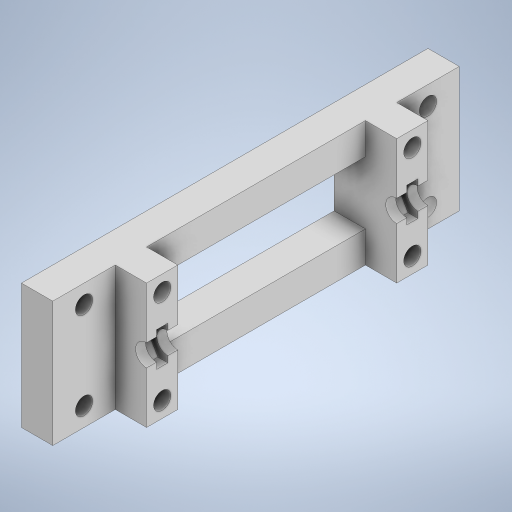
# Autodesk Inventor part: MotorDifferentialMountingBracket
Saved by Autodesk Inventor 2023 (Build 270158000, 158)
## iProperties
Created: 2023-03-28
Part Number: MotorDifferentialMountingBracket
Material: Generic
Document SubType Name: Modeling
Designer: Nathann
Density: 1 g/cm^3
Appearance: Default
Author: Nathann
Autodesk Inventor part; units mm, degrees
ref_plane "YZ Plane" through (0, 0, 0) normal (1, 0, 0) x (0, 1, 0)
ref_plane "XZ Plane" through (0, 0, 0) normal (0, 1, 0) x (-1, 0, 0)
ref_plane "XY Plane" through (0, 0, 0) normal (0, 0, 1) x (1, 0, 0)
sketch "Sketch1" plane through (0, 0, 0) normal (0, 1, 0) x (-1, 0, 0)
  line L0 (0, 0) -> (-5, 0)
  line L1 (-5, 0) -> (-5, 45)
  line L2 (-5, 45) -> (0, 45)
  line L3 (0, 45) -> (0, 0)
  line L4 (-5, 45) -> (-20, 45)
  line L5 (-20, 45) -> (-20, 40)
  line L6 (-20, 40) -> (-5, 40)
  line L7 (-5, 40) -> (-5, 45)
  line L8 (-5, 0) -> (-20, 0)
  line L9 (-20, 0) -> (-20, 5)
  line L10 (-20, 5) -> (-5, 5)
  line L11 (-5, 5) -> (-5, 0)
  point P0 (-5, 40)
  point P1 (-5, 5)
  dimension "d0" = 5
  dimension "d1" = 5
  dimension "d2" = 5
  dimension "d3" = 15
  dimension "d4" = 15
  dimension "d5" = 35
  constraints: 24 end point, 6 parallel, 3 horizontal, 3 perpendicular, 1 point on line
  measures "d0" distance between parallel lines of L3 L1
  measures "d1" distance between parallel lines of L6 L4
  measures "d2" distance between parallel lines of L8 L10
  measures "d3" distance between parallel lines of L5 L1
  measures "d4" distance between parallel lines of L1 L9
  measures "d5" distance between parallel lines of L10 L6
extrude "Extrusion1" add sketch "Sketch1" along normal blind 20
sketch "Sketch2" plane through (0, 0, 45) normal (0, 0, 1) x (1, 0, 0)
  circle A0 centre (10, 10) radius 1.75
  line L0 (20, 0) -> (20, 20) projected
  line L1 (20, 0) -> (10, 0)
  line L2 (10, 0) -> (10, 20)
  line L3 (10, 20) -> (20, 20)
  line L4 (20, 20) -> (20, 0)
  line L5 (0, 0) -> (20, 0) projected
  dimension "d8" = 10
  dimension "d9" = 10
  dimension "d10" = 10
  dimension "d11" = 3.5
  constraints: 8 end point, 2 parallel, 1 centre point, 1 horizontal, 1 perpendicular
  measures "d8" distance between parallel lines of L0 L2
  measures "d9" distance from line of L0 A0.centre
  measures "d10" distance from line of L5 A0.centre
  measures "d11" diameter of A0
extrude "Extrusion2" cut sketch "Sketch2" against normal blind 200
sketch "Sketch3" plane through (0, 0, 0) normal (-1, 0, 0) x (0, 0, 1)
  line L0 (5, 0) -> (5, 20) projected
  line L1 (40, 0) -> (40, 20) projected
  line L2 (5, 15) -> (40, 15)
  line L3 (40, 15) -> (40, 5)
  line L4 (40, 5) -> (5, 5)
  line L5 (5, 5) -> (5, 15)
  line L6 (0, 20) -> (45, 20) projected
  line L7 (0, 0) -> (45, 0) projected
  point P0 (5, 5)
  dimension "d14" = 5
  dimension "d15" = 5
  constraints: 8 end point, 2 parallel, 2 point on line, 1 horizontal, 1 perpendicular
  measures "d14" distance between parallel lines of L6 L2
  measures "d15" distance between parallel lines of L7 L4
extrude "Extrusion3" cut sketch "Sketch3" against normal blind 20 contours L0 L2 L1 L4
sketch "Sketch4" plane through (0, 0, 0) normal (-1, 0, 0) x (0, 0, 1)
  line L0 (45, 0) -> (45, 20) projected
  line L1 (45, 20) -> (55, 20)
  line L2 (55, 20) -> (55, 0)
  line L3 (55, 0) -> (45, 0)
  line L4 (45, 0) -> (45, 20)
  line L5 (0, 20) -> (0, 11.75) projected
  line L6 (0, 20) -> (-10, 20)
  line L7 (-10, 20) -> (-10, 0)
  line L8 (-10, 0) -> (0, 0)
  line L9 (0, 0) -> (0, 20)
  circle A0 centre (50, 3) radius 1.375
  circle A1 centre (50, 17) radius 1.375
  circle A2 centre (-5, 17) radius 1.375
  circle A3 centre (-5, 3) radius 1.375
  point P0 (0, 0)
  point P1 (50, 20)
  dimension "d18" = 10
  dimension "d19" = 10
  dimension "d20" = 3
  dimension "d21" = 3
  dimension "d22" = 5
  dimension "d23" = 5
  dimension "d24" = 5
  dimension "d25" = 5
  dimension "d26" = 3
  dimension "d27" = 3
  dimension "d28" = 2.75
  dimension "d29" = 2.75
  dimension "d30" = 2.75
  dimension "d31" = 2.75
  constraints: 16 end point, 4 centre point, 4 parallel, 2 horizontal, 2 perpendicular, 1 midpoint, 1 point on line
  measures "d18" distance between parallel lines of L0 L2
  measures "d19" distance between parallel lines of L7 L9
  measures "d20" distance from line of L3 A0.centre
  measures "d21" distance of point (50, 20) A1.centre
  measures "d22" distance from line of L2 A0.centre
  measures "d23" distance from line of L2 A1.centre
  measures "d24" distance from line of L7 A2.centre
  measures "d25" distance from line of L7 A3.centre
  measures "d26" distance from line of L8 A3.centre
  measures "d27" distance from line of L6 A2.centre
  measures "d28" diameter of A0
  measures "d29" diameter of A1
  measures "d30" diameter of A2
  measures "d31" diameter of A3
extrude "Extrusion4" add sketch "Sketch4" against normal blind 5
sketch "Sketch5" plane through (10, 11.75, 45) normal (1, 0, 0) x (0, 0, -1)
  circle A0 centre (42.5, 5.75) radius 1.375
  circle A1 centre (42.5, -9.25) radius 1.375
  circle A2 centre (2.5, 5.75) radius 1.375
  circle A3 centre (2.5, -9.25) radius 1.375
  line L0 (40, 8.25) -> (45, 8.25) projected
  line L1 (45, 8.25) -> (45, 0) projected
  line L2 (45, -3.5) -> (45, -11.75) projected
  line L3 (45, -11.75) -> (40, -11.75) projected
  line L4 (5, -11.75) -> (0, -11.75) projected
  line L5 (0, -11.75) -> (0, -3.5) projected
  line L6 (0, 0) -> (0, 8.25) projected
  line L7 (0, 8.25) -> (5, 8.25) projected
  dimension "d34" = 2.5
  dimension "d35" = 2.5
  dimension "d36" = 2.5
  dimension "d37" = 2.5
  dimension "d38" = 2.5
  dimension "d39" = 2.5
  dimension "d40" = 2.5
  dimension "d41" = 2.5
  dimension "d42" = 2.75
  dimension "d43" = 2.75
  dimension "d44" = 2.75
  dimension "d45" = 2.75
  constraints: 4 centre point
  measures "d34" distance from line of L0 A0.centre
  measures "d35" distance from line of L1 A0.centre
  measures "d36" distance from line of L2 A1.centre
  measures "d37" distance from line of L3 A1.centre
  measures "d38" distance from line of L4 A3.centre
  measures "d39" distance from line of L5 A3.centre
  measures "d40" distance from line of L6 A2.centre
  measures "d41" distance from line of L7 A2.centre
  measures "d42" diameter of A2
  measures "d43" diameter of A3
  measures "d44" diameter of A0
  measures "d45" diameter of A1
extrude "Extrusion5" cut sketch "Sketch5" against normal blind 15
sketch "Sketch6" plane through (0, 0, 55) normal (-1, 0, 0) x (0, 0, 1)
  circle A0 centre (-12.5, 17.5) radius 1.375 projected
  circle A1 centre (-12.5, 17.5) radius 2
  circle A2 centre (-12.5, 2.5) radius 1.375 projected
  circle A3 centre (-12.5, 2.5) radius 2
  circle A4 centre (-52.5, 2.5) radius 1.375 projected
  circle A5 centre (-52.5, 2.5) radius 2
  circle A6 centre (-52.5, 17.5) radius 1.375 projected
  circle A7 centre (-52.5, 17.5) radius 2
  point P0 (-55, 0)
  dimension "d48" = 4
  dimension "d49" = 4
  dimension "d50" = 4
  dimension "d51" = 4
  constraints: 4 centre point, 4 coincident
  measures "d48" diameter of A1
  measures "d49" diameter of A3
  measures "d50" diameter of A5
  measures "d51" diameter of A7
extrude "Extrusion6" cut sketch "Sketch6" against normal blind 5 contours A0 | A1 | A2 | A3 | A4 | A5 | A6 | A7
ref_plane "Work Plane1" through (10, 0, 42.5) normal (0, 0, -1) x (-1, 0, 0)
sketch "Sketch7" plane through (10, 0, 42.5) normal (0, 0, -1) x (-1, 0, 0)
  line L0 (-3.1754, 10) -> (-1.5877, 12.75)
  line L1 (-1.5877, 12.75) -> (1.5877, 12.75)
  line L2 (1.5877, 12.75) -> (3.1754, 10)
  line L3 (3.1754, 10) -> (1.5877, 7.25)
  line L4 (1.5877, 7.25) -> (-1.5877, 7.25)
  line L5 (-1.5877, 7.25) -> (-3.1754, 10)
  line L6 (0, 11.75) -> (0, 20) projected
  line L7 (5, 20) -> (0, 20) projected
  line L8 (5, 0) -> (0, 0) projected
  point P0 (10, 0)
  point P1 (0, 10)
  dimension "d54" = 2.75
  dimension "d55" = 0
  dimension "d56" = 10
  dimension "d57" = 20
  constraints: 12 end point, 1 horizontal alignment, 13 other
  measures "d54" distance from line of L1 point (0, 10)
  measures "d55" distance from line of L6 point (0, 10)
  measures "d56" distance from line of L7 point (0, 10)
  measures "d57" distance between parallel lines of L7 L8
extrude "Extrusion7" cut sketch "Sketch7" along normal mid plane 1.8
ref_plane "Work Plane2" through (0, 0, 22.5) normal (0, 0, 1) x (1, 0, 0)
mirror "Mirror1" about plane through (0, 0, 22.5) normal (0, 0, 1) of "Extrusion7"
equation "\"d14\" = d15"
equation "\"d19\" = d18"
equation "\"d20\" = d21"
equation "\"d24\" = d23"
equation "\"d25\" = d22"
equation "\"d26\" = d20"
equation "\"d27\" = d21"
equation "\"d34\" = d35"
equation "\"d37\" = d34"
equation "\"d38\" = d34"
equation "\"d39\" = d36"
equation "\"d40\" = d39"
equation "\"d41\" = d34"
equation "\"d44\" = d42"
equation "\"d45\" = d43"
equation "\"d49\" = d48"
equation "\"d50\" = d49"
equation "\"d51\" = d48"
body "Solid1"
